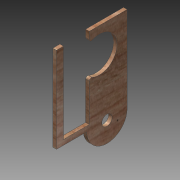
# Autodesk Inventor part: houder
Saved by Autodesk Inventor 2015 (Build 190159000, 159)
## iProperties
Created: 2015-12-31
Part Number: houder
Material: Generic
Document SubType Name: Modeling
Designer: david
Density: 1 g/cm^3
Appearance: Birch - Natural Polished
Author: david
Autodesk Inventor part; units mm, degrees
ref_plane "YZ Plane" through (0, 0, 0) normal (1, 0, 0) x (0, 1, 0)
ref_plane "XZ Plane" through (0, 0, 0) normal (0, 1, 0) x (-1, 0, 0)
ref_plane "XY Plane" through (0, 0, 0) normal (0, 0, 1) x (1, 0, 0)
sketch "Sketch1" plane through (0, 0, 0) normal (1, 0, 0) x (0, 1, 0)
  line L0 (-20, -30) -> (20, -30)
  line L1 (20, -30) -> (20, 30)
  line L2 (20, 30) -> (-20, 30)
  line L3 (-20, 30) -> (-20, -30)
  line L4 (-20, -30) -> (20, 30) construction
  line L5 (20, -30) -> (-20, 30) construction
  circle A0 centre (0, -30) radius 20
  point P0 (0, 0)
  dimension "d0" = 40
  dimension "d1" = 60
  constraints: 12 end point, 3 midpoint, 2 parallel, 1 horizontal, 1 horizontal alignment, 1 perpendicular, 2 other
  measures "d0" distance of L2.end L1.end
  measures "d1" distance of L1.end L0.end
extrude "Extrusion1" add sketch "Sketch1" along normal blind 3.6
sketch "Sketch4" plane through (3.6, 0, 0) normal (1, 0, 0) x (0, 0, -1)
  line L0 (30, 20) -> (-55, 20)
  line L1 (-55, 20) -> (-55, -50)
  line L2 (-55, -50) -> (30, -50)
  line L3 (30, -50) -> (30, 20)
  dimension "d40" = 85
  dimension "d41" = 70
  constraints: 8 end point, 2 parallel, 1 horizontal, 1 perpendicular
  measures "d40" distance of L2.end L1.end
  measures "d41" distance of L1.end L0.end
extrude "Extrusion4" add sketch "Sketch4" against normal blind 3.6
sketch "Sketch2" plane through (0, 0, 0) normal (-1, 0, 0) x (0, 0, 1)
  arc A0 (-30, 20) -> (-30, -20) centre (-30, 0) ccw projected
  circle A1 centre (-30, 0) radius 5.15
  point P0 (0, 0)
  dimension "d4" = 10.3
  constraints: 1 centre point, 1 coincident
  measures "d4" diameter of A1
extrude "Extrusion2" cut sketch "Sketch2" against normal blind 4
sketch "Sketch6" plane through (0, 0, 0) normal (-1, 0, 0) x (0, 0, 1)
  line L0 (55, -50) -> (55, 20) projected
  line L1 (55, -43) -> (-25, -43)
  line L2 (-25, -43) -> (-25, -17.5)
  line L3 (-25, -17.5) -> (55, -17.5)
  line L4 (55, -17.5) -> (55, -43)
  circle A0 centre (30, -7.5) radius 17.5
  line L5 (-30, 20) -> (55, 20) projected
  line L6 (55, -50) -> (-30, -50) projected
  point P0 (0, 0)
  dimension "d42" = 80
  dimension "d43" = 25.5
  dimension "d44" = 35
  dimension "d45" = 25
  dimension "d46" = 27.5
  dimension "d50" = 7
  constraints: 8 end point, 2 parallel, 1 centre point, 1 horizontal, 1 perpendicular, 1 point on line
  measures "d42" distance of L2.end L3.end
  measures "d43" distance of L1.end L2.end
  measures "d44" diameter of A0
  measures "d45" distance from line of L0 A0.centre
  measures "d46" distance from line of L5 A0.centre
  measures "d50" distance between parallel lines of L6 L1
extrude "Extrusion6" cut sketch "Sketch6" against normal blind 10
fillet "Fillet2" radius 2 2 edges at (1.8, -17.5, 15.6386) (1.8, -17.5, 44.3614)
body "Solid1"
